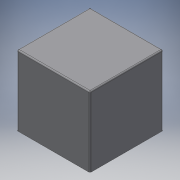
# Autodesk Inventor part: raspberry_box
Saved by Autodesk Inventor 2019 (Build 230136000, 136)
## iProperties
Created: 2022-12-05
Part Number: raspberry_box
Material: S235JR
Document SubType Name: Modellieren
Designer: Damiano Pezzè
Density: 1 g/cm^3
Appearance: Vorgabe
Author: Damiano Pezzè
Autodesk Inventor part; units mm, degrees
ref_plane "YZ Ebene" through (0, 0, 0) normal (1, 0, 0) x (0, 1, 0)
ref_plane "XZ Ebene" through (0, 0, 0) normal (0, 1, 0) x (-1, 0, 0)
ref_plane "XY Ebene" through (0, 0, 0) normal (0, 0, 1) x (1, 0, 0)
sketch "Sketch20" plane through (0, 0, 0) normal (0, 1, 0) x (-1, 0, 0)
  line L0 (0, 0) -> (120, 0)
  line L1 (120, 0) -> (120, -120)
  line L2 (120, -120) -> (0, -120)
  line L3 (0, -120) -> (0, 0)
  dimension "d58" = 120
  dimension "d59" = 120
  constraints: 8 end point, 2 parallel, 1 horizontal, 1 perpendicular
  measures "d58" distance of L1.end L2.end
  measures "d59" distance of L0.end L1.end
extrude "Extrusion8" add sketch "Sketch20" along normal blind 115
sketch "Sketch21" plane through (0, 0, 0) normal (0, -1, 0) x (1, 0, 0)
  line L0 (-5, -5) -> (-115, -5)
  line L1 (-115, -5) -> (-115, -115)
  line L2 (-115, -115) -> (-5, -115)
  line L3 (-5, -115) -> (-5, -5)
  line L4 (0, -120) -> (0, 0) projected
  line L5 (0, 0) -> (-120, 0) projected
  dimension "d62" = 110
  dimension "d63" = 110
  dimension "d64" = 5
  dimension "d65" = 5
  constraints: 8 end point, 2 parallel, 1 horizontal, 1 perpendicular
  measures "d62" distance of L2.end L1.end
  measures "d63" distance of L1.end L0.end
  measures "d64" distance between parallel lines of L4 L3
  measures "d65" distance between parallel lines of L5 L0
extrude "Extrusion9" cut sketch "Sketch21" against normal blind 110
sketch "Sketch22" plane through (0, 110, 0) normal (0, -1, 0) x (1, 0, 0)
  line L0 (-115, -115) -> (-115, -5) projected
  line L1 (-115, -5) -> (-5, -5) projected
  circle A0 centre (-105, -59) radius 5
  circle A1 centre (-105, -10) radius 5
  circle A2 centre (-47, -59) radius 5
  circle A3 centre (-47, -10) radius 5
  point P0 (0, 0)
  dimension "d68" = 10
  dimension "d69" = 5
  dimension "d70" = 49
  dimension "d71" = 58
  dimension "d72" = 10
  dimension "d73" = 10
  dimension "d74" = 10
  dimension "d75" = 10
  constraints: 4 centre point, 4 coincident
  measures "d68" distance from line of L0 point (-105, -10)
  measures "d69" distance from line of L1 point (-105, -10)
  measures "d70" distance of point (-105, -10) point (-105, -59)
  measures "d71" distance of point (-105, -59) point (-47, -59)
  measures "d72" diameter of A0
  measures "d73" diameter of A1
  measures "d74" diameter of A2
  measures "d75" diameter of A3
extrude "Extrusion10" add sketch "Sketch22" along normal blind 5
sketch "Sketch23" plane through (-105, 105, -59) normal (0, -1, 0) x (1, 0, 0)
  circle A0 centre (0, 49) radius 5 projected
  circle A1 centre (58, 0) radius 5 projected
  circle A2 centre (58, 49) radius 5 projected
  point P0 (105, 59)
  point P1 (0, 0)
  point P2 (0, 54)
  point P3 (58, 54)
  constraints: 3 coincident, 2 vertical alignment
hole "Hole2" at (-105, 105, -59) at (-105, 105, -10) at (-47, 105, -59) at (-47, 105, -10) direction (0, 1, 0) diameter 1.57 depth 5
fillet "Fillet5" radius 2 8 edges at (0, 57.5, 0) (-60, 115, 0) (0, 115, -60) (0, 57.5, -120) (-60, 115, -120) (-120, 115, -60) (-120, 57.5, -120) (-120, 57.5, 0)
sketch "Sketch24" plane through (0, 0, 0) normal (0, -1, 0) x (1, 0, 0)
  line L0 (-115, -5) -> (-105, -5) projected
  circle A0 centre (-115, -5) radius 5
  line L1 (-115, -5) -> (-5, -5) projected
  circle A1 centre (-5, -5) radius 5
  line L2 (-5, -5) -> (-5, -115) projected
  circle A2 centre (-5, -115) radius 5
  line L3 (-5, -115) -> (-115, -115) projected
  circle A3 centre (-115, -115) radius 5
  line L4 (-115, -115) -> (-115, -5) projected
  circle A4 centre (-115, -60) radius 5
  circle A5 centre (-5, -60) radius 5
  circle A6 centre (-60, -115) radius 5
  circle A7 centre (-60, -5) radius 5
  point P0 (0, 0)
  dimension "d86" = 10
  dimension "d87" = 10
  dimension "d88" = 10
  dimension "d89" = 10
  dimension "d90" = 10
  dimension "d91" = 10
  dimension "d92" = 10
  dimension "d93" = 10
  constraints: 8 centre point, 3 midpoint
  measures "d86" diameter of A0
  measures "d87" diameter of A1
  measures "d88" diameter of A2
  measures "d89" diameter of A3
  measures "d90" diameter of A4
  measures "d91" diameter of A5
  measures "d92" diameter of A6
  measures "d93" diameter of A7
extrude "Extrusion11" add sketch "Sketch24" against normal blind 10 contours L4 A0 L0 | L0 A0 L4 | A4 L4 | L4 A4 | A7 L1 | L1 A7 | L4 L3 A3 | A3 L3 L4 | A1 L2 L1 | L1 L2 A1 | A6 L3 | L3 A6 | A5 L2 | L2 A5 | L3 L2 A2 | A2 L2 L3
fillet "Fillet6" radius 2 8 edges at (-110, 10, -60) (-111.4645, 10, -111.4645) (-60, 10, -110) (-8.5355, 10, -111.4645) (-10, 10, -60) (-111.4645, 10, -8.5355) (-60, 10, -10) (-8.5355, 10, -8.5355)
sketch "Sketch25" plane through (0, 0, 0) normal (0, -1, 0) x (1, 0, 0)
  line L0 (-5, -8) -> (-5, -5) projected
  line L1 (-5, -63) -> (-5, -57) projected
  line L2 (-5, -115) -> (-115, -115) projected
  line L3 (-57, -5) -> (-63, -5) projected
  line L4 (-115, -57) -> (-115, -63) projected
  line L5 (-112, -5) -> (-115, -5) projected
  point P0 (0, 0)
  point P1 (-5, -60)
  point P2 (-60, -5)
  point P3 (-60, -115)
  point P4 (-115, -60)
  constraints: 4 midpoint, 1 coincident
hole "Hole3" at (-5, 0, -5) at (-5, 0, -60) at (-5, 0, -115) at (-60, 0, -5) at (-60, 0, -115) at (-115, 0, -60) at (-115, 0, -5) at (-115, 0, -115) direction (0, 1, 0) diameter 2.46 depth 8.8 thread size "M3x0.5" class "6H" standard "ISO Metric profile"
body "Solid1"
